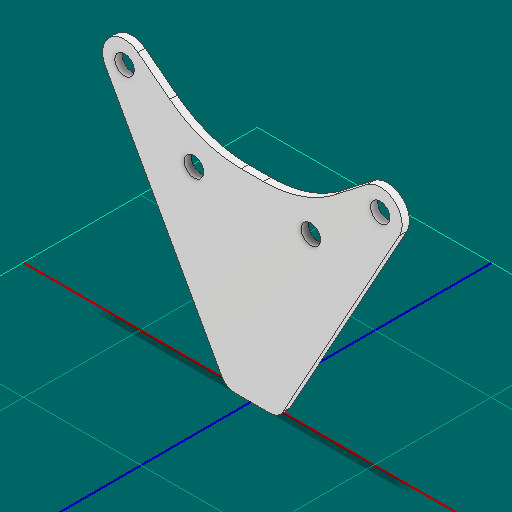
# Autodesk Inventor part: Hook Gussett
Saved by Autodesk Inventor 2025 (Build 290162000, 162)
## iProperties
Created: 2024-10-13
Part Number: Hook Gussett
Material: Acetal Resin, White
Document SubType Name: Modeling
Designer: Averey Ku
Density: 1.425 g/cm^3
Appearance: Smooth - White
Author: Averey Ku
Autodesk Inventor part; units mm, degrees
ref_plane "YZ Plane" through (0, 0, 0) normal (1, 0, 0) x (0, 1, 0)
ref_plane "XZ Plane" through (0, 0, 0) normal (0, 1, 0) x (-1, 0, 0)
ref_plane "XY Plane" through (0, 0, 0) normal (0, 0, 1) x (1, 0, 0)
sketch "Sketch1" plane through (0, 0, 0) normal (0, 0, 1) x (1, 0, 0)
  circle A0 centre (13.2036, 20.3187) radius 2.0955
  circle A1 centre (-12.1964, 20.3187) radius 2.0955
  line L0 (2.9057, 25.0812) -> (-1.8984, 25.0812)
  line L1 (4.3471, -17.7813) -> (-3.3398, -17.7813)
  arc A2 (4.3471, -17.7813) -> (7.3873, -15.5216) centre (4.3471, -14.6063) ccw
  arc A3 (-6.38, -15.5216) -> (-3.3398, -17.7813) centre (-3.3398, -14.6063) ccw
  circle A4 centre (-27.2689, 31.9687) radius 2.0955
  arc A5 (-24.3564, 35.7368) -> (-31.437, 29.6649) centre (-27.2689, 31.9687) ccw
  line L2 (-31.437, 29.6649) -> (-6.1186, -16.1422)
  arc A6 (32.4443, 29.6649) -> (25.3636, 35.7368) centre (28.2761, 31.9687) ccw
  circle A7 centre (28.2761, 31.9687) radius 2.0955
  line L3 (32.4443, 29.6649) -> (7.1258, -16.1422)
  line L4 (-24.3564, 35.7368) -> (-17.4317, 30.3845)
  line L5 (25.3636, 35.7368) -> (18.439, 30.3845)
  arc A8 (-17.4317, 30.3845) -> (-1.8984, 25.0812) centre (-1.8984, 50.4812) ccw
  arc A9 (2.9057, 25.0812) -> (18.439, 30.3845) centre (2.9057, 50.4812) ccw
  point P0 (0, 0)
  point P1 (-12.1964, 25.0812)
  point P2 (17.4758, 18.214)
  point P3 (-16.4686, 18.214)
  dimension "d1" = 3.175
  dimension "d8" = 4.191
  dimension "d9" = 4.191
  dimension "d13" = 4.191
  dimension "d14" = 9.525
  dimension "d15" = 9.525
  dimension "d16" = 4.191
  dimension "d17" = 25.4
  constraints: 14 point on circle, 12 end point, 12 tangent, 10 centre point, 2 coincident, 2 equal radius, 2 horizontal, 2 other
  measures "d1" radius of A2
  measures "d8" diameter of A1
  measures "d9" diameter of A0
  measures "d13" diameter of A4
  measures "d14" diameter of A5
  measures "d15" diameter of A6
  measures "d16" diameter of A7
  measures "d17" radius of A8
extrude "Extrusion1" add sketch "Sketch1" along normal blind 1.5875
body "Solid1"
